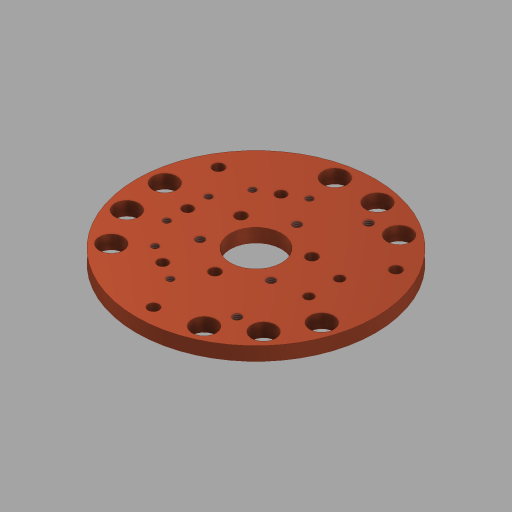
# Autodesk Inventor part: TopRing-2023-1
Saved by Autodesk Inventor 2024 (Build 280153020, 153B)
## iProperties
Created: 2018-11-20
Part Number: TopRing-2023-1
Material: Copper
Document SubType Name: Modeling
Designer: schanen
Density: 8.94 g/cm^3
Appearance: Copper - Satin
Mass: 121.653 g
Surface Area: 89.8116 cm^2
Volume: 13.6077 cm^3
Author: schanen
Autodesk Inventor part; units mm, degrees
ref_plane "YZ Plane" through (0, 0, 0) normal (1, 0, 0) x (0, 1, 0)
ref_plane "XZ Plane" through (0, 0, 0) normal (0, 1, 0) x (-1, 0, 0)
ref_plane "XY Plane" through (0, 0, 0) normal (0, 0, 1) x (1, 0, 0)
sketch "Sketch1" plane through (0, 0, 0) normal (0, 1, 0) x (-1, 0, 0)
  circle A0 centre (0, 0) radius 35
  circle A1 centre (0, 0) radius 7.5
  dimension "d0" = 70
  dimension "d129" = 15
  constraints: 2 centre point, 2 coincident
  measures "d0" diameter of A0
  measures "d129" diameter of A1
extrude "Extrusion1" add sketch "Sketch1" along normal blind 4
sketch "Sketch2" plane through (0, 4, 0) normal (0, 1, 0) x (1, 0, 0)
  circle A0 centre (0, 0) radius 30 construction
  point P0 (0, -30)
  point P1 (-25.9808, 15)
  point P2 (25.9808, 15)
  dimension "d130" = 60
  dimension "d131" = 120
  dimension "d132" = 120
  constraints: 3 point on circle, 1 centre point, 1 coincident, 1 vertical alignment
  measures "d130" diameter of A0
hole "Hole1" at (-25.9808, 4, -15) at (25.9808, 4, -15) at (0, 4, 30) direction (0, -1, 0) diameter 3.2 end through all
sketch "Sketch15" plane through (0, 4, 0) normal (0, 1, 0) x (1, 0, 0)
  circle A0 centre (0, 0) radius 30 construction
  circle A1 centre (0, -30) radius 1.6 projected
  line L0 (0, 0) -> (0, -30) construction
  point P0 (12.2021, -27.4064)
  point P1 (0, -15)
  point P2 (17.6336, 24.2705)
  point P3 (-29.8357, 3.1359)
  point P4 (-22.2943, -20.0739)
  point P5 (28.5317, -9.2705)
  point P6 (-6.2374, 29.3444)
  dimension "d137" = 60
  dimension "d138" = 24
  dimension "d141" = 360
  dimension "d143" = 48
  dimension "d146" = 360
  constraints: 2 end point, 2 point on circle, 1 centre point, 1 coincident, 1 midpoint, 1 vertical, 8 other
  measures "d137" diameter of A0
hole "Hole13" at (12.2021, 4, 27.4064) at (17.6336, 4, -24.2705) at (-29.8357, 4, -3.1359) at (-22.2943, 4, 20.0739) at (28.5317, 4, 9.2705) at (-6.2374, 4, -29.3444) direction (0, -1, 0) diameter 7 end through all
sketch "Sketch16" plane through (0, 4, 0) normal (0, 1, 0) x (1, 0, 0)
  circle A0 centre (0, 0) radius 12 construction
  point P0 (0, -12)
  point P1 (-10.3923, 6)
  point P2 (10.3923, 6)
  dimension "d155" = 24
  dimension "d156" = 120
  dimension "d157" = 120
  constraints: 3 point on circle, 1 centre point, 1 coincident, 1 vertical alignment
  measures "d155" diameter of A0
hole "Hole14" at (0, 4, 12) at (-10.3923, 4, -6) at (10.3923, 4, -6) direction (0, -1, 0) diameter 3.2 end through all
sketch "Sketch17" plane through (0, 4, 0) normal (0, 1, 0) x (1, 0, 0)
  circle A0 centre (0, 0) radius 12 construction
  point P0 (0, 12)
  point P1 (-10.3923, -6)
  point P2 (10.3923, -6)
  dimension "d165" = 24
  dimension "d166" = 120
  dimension "d167" = 120
  constraints: 3 point on circle, 1 centre point, 1 coincident, 1 vertical alignment
  measures "d165" diameter of A0
hole "Hole15" at (0, 4, -12) at (-10.3923, 4, 6) at (10.3923, 4, 6) direction (0, -1, 0) diameter 2.459 end through all thread size "M3x0.5" class "6H" standard "ANSI Metric M Profile"
sketch "Sketch18" plane through (0, 4, 0) normal (0, 1, 0) x (1, 0, 0)
  point P0 (0, 0)
  point P1 (20, 4.5)
  point P2 (20, -4.5)
  dimension "d175" = 9
  dimension "d176" = 4.5
  dimension "d177" = 20
  measures "d175" distance of point (20, -4.5) point (20, 4.5)
  measures "d176" vertical distance of point (0, 0) point (20, -4.5)
  measures "d177" horizontal distance of point (0, 0) point (20, -4.5)
hole "Hole16" at (20, 4, -4.5) at (20, 4, 4.5) direction (0, -1, 0) diameter 2.7 end through all
sketch "Sketch19" plane through (0, 4, 0) normal (0, 1, 0) x (1, 0, 0)
  circle A0 centre (0, 0) radius 20 construction
  point P0 (-20, 0)
  point P1 (-10, 17.3205)
  point P2 (-10, -17.3205)
  dimension "d185" = 40
  dimension "d186" = 60
  dimension "d187" = 60
  constraints: 3 point on circle, 1 centre point, 1 coincident, 1 horizontal alignment
  measures "d185" diameter of A0
hole "Hole17" at (-20, 4, 0) at (-10, 4, -17.3205) at (-10, 4, 17.3205) direction (0, -1, 0) diameter 3 end through all
sketch "Sketch20" plane through (0, 4, 0) normal (0, 1, 0) x (1, 0, 0)
  circle A0 centre (-20, 0) radius 1.5 projected
  point P0 (0, 0)
  point P1 (-20, 6.1)
  point P2 (-20, -6.1)
  point P3 (-4.7172, -20.3705)
  point P4 (-15.2828, -14.2705)
  point P5 (-15.2828, 14.2705)
  point P6 (-4.7172, 20.3705)
  point P7 (0, 0)
  dimension "d195" = 12.2
  dimension "d196" = 6.1
  dimension "d199" = 60
  dimension "d203" = 60
  constraints: 2 vertical alignment, 1 coincident, 6 other
  measures "d195" distance of point (-20, 6.1) point (-20, -6.1)
  measures "d196" distance of A0.centre point (-20, -6.1)
hole "Hole18" at (-20, 4, -6.1) at (-20, 4, 6.1) at (-4.7172, 4, 20.3705) at (-15.2828, 4, 14.2705) at (-15.2828, 4, -14.2705) at (-4.7172, 4, -20.3705) direction (0, -1, 0) diameter 2.013 end through all thread size "M2.5x0.45" class "6H" standard "ANSI Metric M Profile"
sketch "Sketch21" plane through (0, 4, 0) normal (0, 1, 0) x (1, 0, 0)
  circle A0 centre (0, 0) radius 25 construction
  circle A1 centre (0, -30) radius 1.6 projected
  point P0 (14.6946, -20.2254)
  point P1 (10.1684, 22.8386)
  dimension "d212" = 50
  dimension "d222" = 120
  dimension "d223" = 36
  constraints: 2 point on circle, 1 centre point, 1 coincident
  measures "d212" diameter of A0
hole "Hole19" at (14.6946, 4, 20.2254) at (10.1684, 4, -22.8386) direction (0, -1, 0) diameter 2.459 end through all thread size "M3x0.5" class "6H" standard "ANSI Metric M Profile"
sketch "Sketch22" plane through (0, 4, 0) normal (0, 1, 0) x (1, 0, 0)
  circle A0 centre (28.5317, -9.2705) radius 3.5 projected
  line L0 (0, 0) -> (28.5317, -9.2705) construction
  circle A1 centre (12.2021, -27.4064) radius 3.5 projected
  line L1 (0, 0) -> (12.2021, -27.4064) construction
  circle A2 centre (0, 0) radius 30 construction
  line L2 (0, 0) -> (22.2943, -20.0739) construction
  dimension "d224" = 48
  dimension "d227" = 24
  constraints: 6 end point, 2 coincident, 2 point on circle, 1 centre point
  measures "d224" angle of L0 L1
  measures "d227" angle of L1 L2
hole "Hole20" at (22.2943, 4, 20.0739) direction (0, -1, 0) diameter 7 end through all
pattern_circular "Circular Pattern5" count 3 over 360 about axis through (0, 0, 0) along (0, 1, 0) of "Hole20"
equation "\"d176\" = 0.5 * d175"
equation "\"d196\" = 0.5 * d195"
equation "\"d227\" = 0.5 * d224"
body "Solid1"
